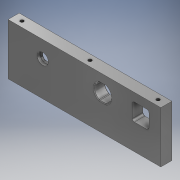
# Autodesk Inventor part: back accses panel
Saved by Autodesk Inventor 2019 (Build 230136000, 136)
## iProperties
Created: 2018-05-03
Part Number: back accses panel
Material: Aluminum 6061
Document SubType Name: Modeling
Designer: SimonD
Density: 2.7 g/cm^3
Appearance: Aluminum - Polished
Author: SimonD
Autodesk Inventor part; units mm, degrees
ref_plane "YZ Plane" through (0, 0, 0) normal (1, 0, 0) x (0, 1, 0)
ref_plane "XZ Plane" through (0, 0, 0) normal (0, 1, 0) x (-1, 0, 0)
ref_plane "XY Plane" through (0, 0, 0) normal (0, 0, 1) x (1, 0, 0)
sketch "Sketch1" plane through (0, 0, 0) normal (0, 0, 1) x (1, 0, 0)
  line L0 (-55, 4) -> (55, 4)
  line L1 (55, 4) -> (55, -4)
  line L2 (55, -4) -> (-55, -4)
  line L3 (-55, -4) -> (-55, 4)
  line L4 (-55, 4) -> (55, -4) construction
  line L5 (55, 4) -> (-55, -4) construction
  point P0 (0, 0)
  dimension "d0" = 110
  dimension "d1" = 8
  constraints: 12 end point, 2 midpoint, 2 parallel, 1 horizontal, 1 perpendicular
  measures "d0" distance of L1.end L2.end
  measures "d1" distance between parallel lines of L2 L0
extrude "Extrusion1" add sketch "Sketch1" along normal blind 37
sketch "Sketch2" plane through (0, 0, 37) normal (0, 0, 1) x (1, 0, 0)
  line L0 (-55, 4) -> (-55, -4) projected
  line L1 (55, -4) -> (55, 4) projected
  point P0 (0, 0)
  point P1 (-49, 0)
  point P2 (0, 0)
  point P3 (49, 0)
  dimension "d4" = 6
  dimension "d5" = 6
  constraints: 1 coincident
  measures "d4" distance from line of point (-49, 0) L0
  measures "d5" distance from line of L1 point (49, 0)
hole "Hole1" at (-49, 0, 37) at (0, 0, 37) at (49, 0, 37) direction (0, 0, -1) diameter 2.459 depth 8 tip angle 118 thread size "M3x0.5" class "6H" standard "ISO Metric profile"
fillet "Fillet1" [suppressed]
sketch "Sketch3" plane through (0, 0, 0) normal (0, 0, -1) x (-1, 0, 0)
  circle A0 centre (-49, 0) radius 1.2295 projected
  circle A1 centre (0, 0) radius 1.2295 projected
  circle A2 centre (49, 0) radius 1.2295 projected
  constraints: 3 coincident
hole "Hole2" at (49, 0, 0) at (0, 0, 0) at (-49, 0, 0) direction (0, 0, 1) diameter 2.459 depth 8 tip angle 118 thread size "M3x0.5" class "6H" standard "ISO Metric profile"
sketch "Sketch6" plane through (-55, -4, 0) normal (0, -1, 0) x (1, 0, 0)
  line L0 (89.5, 18.5) -> (101.5, 18.5)
  line L1 (101.5, 18.5) -> (101.5, 31)
  line L2 (101.5, 31) -> (89.5, 31)
  line L3 (89.5, 31) -> (89.5, 18.5)
  line L4 (110, 0) -> (110, 37) projected
  line L5 (110, 0) -> (0, 0) projected
  line L6 (0, 37) -> (110, 37) projected
  point P0 (55, 0)
  dimension "d34" = 8.5
  dimension "d35" = 12
  dimension "d61" = 6
  dimension "d62" = 12.5
  constraints: 8 end point, 2 parallel, 1 horizontal, 1 perpendicular
  measures "d34" distance between parallel lines of L4 L1
  measures "d35" distance between parallel lines of L3 L1
  measures "d61" distance between parallel lines of L2 L6
  measures "d62" distance between parallel lines of L0 L2
extrude "Extrusion3" cut sketch "Sketch6" against normal blind 10
fillet "Fillet2" radius 1.5 4 edges at (34.5, 0, 31) (46.5, 0, 31) (46.5, 0, 18.5) (34.5, 0, 18.5)
sketch "Sketch7" plane through (-55, 4, 0) normal (0, 1, 0) x (1, 0, 0)
  circle A0 centre (25, -25) radius 4
  line L0 (110, -37) -> (0, -37) projected
  line L1 (110, 0) -> (110, -37) projected
  point P0 (55, 0)
  dimension "d44" = 8
  dimension "d45" = 12
  dimension "d46" = 85
  constraints: 1 centre point
  measures "d44" diameter of A0
  measures "d45" distance from line of A0.centre L0
  measures "d46" distance from line of A0.centre L1
extrude "Extrusion4" cut sketch "Sketch7" against normal blind 10
sketch "Sketch9" plane through (-55, 4, 0) normal (0, 1, 0) x (1, 0, 0)
  line L0 (32.5, -32.5) -> (17.5, -32.5)
  line L1 (17.5, -32.5) -> (17.5, -17.5)
  line L2 (17.5, -17.5) -> (32.5, -17.5)
  line L3 (32.5, -17.5) -> (32.5, -32.5)
  circle A0 centre (25, -25) radius 4 projected
  line L4 (32.5, -32.5) -> (17.5, -17.5) construction
  line L5 (17.5, -32.5) -> (32.5, -17.5) construction
  point P0 (55, 0)
  dimension "d52" = 15
  dimension "d53" = 15
  constraints: 12 end point, 2 midpoint, 2 parallel, 1 horizontal, 1 perpendicular
  measures "d52" distance of L1.end L2.end
  measures "d53" distance between parallel lines of L2 L0
extrude "Extrusion6" cut sketch "Sketch9" against normal blind 6
fillet "Fillet3" radius 2 4 edges at (-22.5, 1, 32.5) (-22.5, 1, 17.5) (-37.5, 1, 17.5) (-37.5, 1, 32.5)
chamfer "Chamfer3" distance 0.5 angle 45 16 edges at (40.5, 4, 31) (34.9393, 4, 30.5607) (34.5, 4, 24.75) (34.9393, 4, 18.9393) (40.5, 4, 18.5) (46.0607, 4, 18.9393) (46.5, 4, 24.75) (46.0607, 4, 30.5607) (-30, 4, 17.5) (-23.0858, 4, 18.0858) (-22.5, 4, 25) (-23.0858, 4, 31.9142) (-30, 4, 32.5) (-36.9142, 4, 31.9142) (-37.5, 4, 25) (-36.9142, 4, 18.0858)
sketch "Sketch10" plane through (-55, 4, 0) normal (0, 1, 0) x (1, 0, 0)
  line L0 (110, 0) -> (110, -37) projected
  line L1 (70.5, -30.6736) -> (65.5, -30.6736)
  line L2 (65.5, -19.3264) -> (70.5, -19.3264)
  line L3 (70.5, -30.6736) -> (65.5, -19.3264) construction
  line L4 (65.5, -30.6736) -> (70.5, -19.3264) construction
  arc A0 (70.5, -30.6736) -> (70.5, -19.3264) centre (68, -25) ccw
  arc A1 (65.5, -19.3264) -> (65.5, -30.6736) centre (68, -25) ccw
  point P0 (55, 0)
  dimension "d70" = 42
  dimension "d74" = 5
  constraints: 8 end point, 4 point on circle, 2 centre point, 2 midpoint, 1 horizontal, 1 parallel
  measures "d70" distance from line of A0.centre L0
  measures "d74" distance of L2.start L2.end
extrude "Extrusion7" cut sketch "Sketch10" against normal blind 10
chamfer "Chamfer4" [suppressed]
fillet "Fillet5" radius 1.5 4 edges at (15.5, 0, 30.6736) (10.5, 0, 30.6736) (15.5, 0, 19.3264) (10.5, 0, 19.3264)
chamfer "Chamfer5" distance 0.5 angle 45 16 edges at (13, 4, 19.3264) (15.5162, 4, 19.369) (19.2, 4, 25) (15.5162, 4, 30.631) (13, 4, 30.6736) (10.4838, 4, 30.631) (6.8, 4, 25) (10.4838, 4, 19.369) (19.2, -4, 25) (15.5162, -4, 19.369) (13, -4, 19.3264) (10.4838, -4, 19.369) (6.8, -4, 25) (10.4838, -4, 30.631) (13, -4, 30.6736) (15.5162, -4, 30.631)
body "Solid1"
